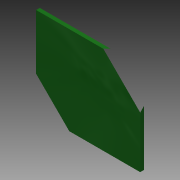
# Autodesk Inventor part: CombinerBoard
Saved by Autodesk Inventor 2014 (Build 180170000, 170)
## iProperties
Created: 2015-04-15
Part Number: CombinerBoard
Material: Generic
Document SubType Name: Modeling
Designer: Owner
Density: 1 g/cm^3
Appearance: Smooth - Dark Forest Green
Author: Owner
Autodesk Inventor part; units mm, degrees
ref_plane "YZ Plane" through (0, 0, 0) normal (1, 0, 0) x (0, 1, 0)
ref_plane "XZ Plane" through (0, 0, 0) normal (0, 1, 0) x (-1, 0, 0)
ref_plane "XY Plane" through (0, 0, 0) normal (0, 0, 1) x (1, 0, 0)
sketch "Sketch1" plane through (0, 0, 0) normal (0, 0, 1) x (1, 0, 0)
  line L0 (15.9308, -19.7489) -> (-31.3132, -19.7489)
  line L1 (-31.3132, -19.7489) -> (-31.3132, 20.3831)
  line L2 (-31.3132, 20.3831) -> (15.9308, 20.3831)
  line L3 (15.9308, 20.3831) -> (15.9308, -19.7489)
  point P0 (0, 0)
  dimension "d0" = 40.132
  dimension "d1" = 47.244
  constraints: 8 end point, 2 parallel, 1 horizontal, 1 perpendicular
  measures "d0" distance of L2.end L0.start
  measures "d1" distance of L1.end L2.end
extrude "Extrusion1" add sketch "Sketch1" along normal blind 1.67
body "Solid1"
